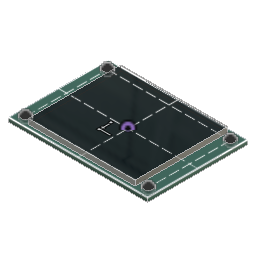
ST7899_240x240_Display v3 (Autodesk Fusion 360 design; units mm, degrees)
Autodesk Fusion 360 part; units mm, degrees
sketch "Sketch1" plane through (0, 0, 0) normal (0, 0, 1) x (1, 0, 0)
  line L0 (-19.5, 14) -> (19.5, 14)
  line L1 (19.5, 14) -> (19.5, -14)
  line L2 (19.5, -14) -> (-19.5, -14)
  line L3 (-19.5, -14) -> (-19.5, 14)
  line L4 (0, 14) -> (0, -14) construction
  line L5 (-19.5, 0) -> (19.5, 0) construction
  circle A0 centre (-17.25, 11.5) radius 1 construction
  circle A1 centre (17.25, 11.5) radius 1 construction
  circle A2 centre (-17.25, -11.5) radius 1 construction
  circle A3 centre (17.25, -11.5) radius 1 construction
  line L6 (-17.25, 11.5) -> (17.25, 11.5) construction
  line L7 (17.25, 11.5) -> (17.25, -11.5) construction
  line L8 (17.25, -11.5) -> (-17.25, -11.5) construction
  line L9 (-17.25, -11.5) -> (-17.25, 11.5) construction
  dimension "d1" = 28
  dimension "d2" = 39
  dimension "d3" = 17.25
  dimension "d4" = 17.25
  dimension "d5" = 11.5
  dimension "d6" = 11.5
  dimension "d7" = 2
  constraint horizontal L0
  constraint vertical L1
  constraint horizontal L2
  constraint vertical L3
  constraint midpoint L0 L4.start
  constraint midpoint L2 L4.end
  constraint midpoint L3 L5.start
  constraint midpoint L1 L5.end
  constraint coincident origin L4
  constraint coincident origin L5
  constraint equal A0 A1
  constraint equal A2 A3
  constraint equal A1 A3
  constraint horizontal L6
  constraint vertical L7
  constraint horizontal L8
  constraint vertical L9
  constraint coincident A0.centre L6.start
  constraint coincident A1.centre L6.end
  constraint coincident A3.centre L7.end
  constraint coincident A2.centre L8.end
  measures "d1" distance of L0.end L1.end
  measures "d2" distance of L0.start L0.end
  measures "d3" distance of origin L9
  measures "d4" distance of origin L7
  measures "d5" distance of origin L6
  measures "d6" distance of origin L8
  measures "d7" diameter of A0
extrude "Extrude1" add sketch "Sketch1" against normal blind 1.2 makes body 1
hole "Hole1" at (-17.25, 11.5, 0) at (17.25, 11.5, 0) at (17.25, -11.5, 0) at (-17.25, -11.5, 0) direction (0, 0, -1) diameter 2 depth 1.2 tip angle 180 bodies 1
sketch "Sketch2" plane through (0, 0, 0) normal (0, 0, 1) x (1, 0, 0)
  line L0 (-15, 13) -> (15, 13)
  line L1 (15, 13) -> (15, -13)
  line L2 (15, -13) -> (-15, -13)
  line L3 (-15, -13) -> (-15, 13)
  line L4 (0, 13) -> (0, -12.6799) construction
  line L5 (-15, 0) -> (15, 0) construction
  dimension "d13" = 26
  dimension "d14" = 30
  constraint horizontal L0
  constraint vertical L1
  constraint horizontal L2
  constraint vertical L3
  constraint midpoint L0 L4.start
  constraint perpendicular L2 L4
  constraint midpoint L3 L5.start
  constraint midpoint L1 L5.end
  constraint coincident L5 origin
  constraint coincident L4 origin
  measures "d13" distance of L0.end L1.end
  measures "d14" distance of L0.start L0.end
extrude "Extrude2" add sketch "Sketch2" along normal blind 1.5 separate body makes body 2
equation "d4 = d3"
equation "d6 = d5"
named bodies: "PCB", "Screen"
